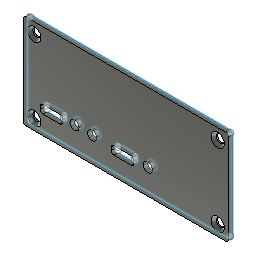
Front Plate (Autodesk Fusion 360 design; units mm, degrees)
Autodesk Fusion 360 part; units mm, degrees
sketch "sketch 658" plane through (0, 0, 0) normal (0, -1, 0) x (1, 0, 0)
  circle A0 centre (8.103, -8.2082) radius 1.7
  arc A1 (-24.375, -7.4644) -> (-23.375, -8.4644) centre (-24.375, -8.4644) cw
  line L0 (-23.375, -8.4644) -> (-23.375, -9.5644)
  arc A2 (-23.375, -9.5644) -> (-24.375, -10.5644) centre (-24.375, -9.5644) cw
  line L1 (-24.375, -10.5644) -> (-30.775, -10.5644)
  arc A3 (-30.775, -10.5644) -> (-31.775, -9.5644) centre (-30.775, -9.5644) cw
  line L2 (-31.775, -9.5644) -> (-31.775, -8.4644)
  arc A4 (-31.775, -8.4644) -> (-30.775, -7.4644) centre (-30.775, -8.4644) cw
  line L3 (-30.775, -7.4644) -> (-24.375, -7.4644)
  line L4 (-4.475, -7.5152) -> (1.925, -7.5152)
  line L5 (-4.475, -7.5152) -> (1.925, -7.5152)
  arc A5 (1.925, -7.5152) -> (2.925, -8.5152) centre (1.925, -8.5152) cw
  line L6 (2.925, -8.5152) -> (2.925, -9.6152)
  arc A6 (2.925, -9.6152) -> (1.925, -10.6152) centre (1.925, -9.6152) cw
  line L7 (1.925, -10.6152) -> (-4.475, -10.6152)
  line L8 (1.925, -10.6152) -> (-4.475, -10.6152)
  arc A7 (-4.475, -10.6152) -> (-5.475, -9.6152) centre (-4.475, -9.6152) cw
  line L9 (-5.475, -9.6152) -> (-5.475, -8.5152)
  arc A8 (-5.475, -8.5152) -> (-4.475, -7.5152) centre (-4.475, -8.5152) cw
  circle A9 centre (-19.0635, -8.2082) radius 1.7
  circle A10 centre (-12.4985, -8.2082) radius 1.7
  arc A11 (-37, 17.5) -> (-38, 16.5) centre (-37, 16.5) ccw
  line L10 (-38, 16.5) -> (-38, -16.5)
  line L11 (-38, 16.5) -> (-38, -16.5)
  arc A12 (-38, -16.5) -> (-37, -17.5) centre (-37, -16.5) ccw
  line L12 (-37, -17.5) -> (37, -17.5)
  line L13 (-37, -17.5) -> (37, -17.5)
  arc A13 (37, -17.5) -> (38, -16.5) centre (37, -16.5) ccw
  line L14 (38, -16.5) -> (38, 16.5)
  line L15 (38, -16.5) -> (38, 16.5)
  arc A14 (38, 16.5) -> (37, 17.5) centre (37, 16.5) ccw
  line L16 (37, 17.5) -> (-37, 17.5)
  line L17 (37, 17.5) -> (-37, 17.5)
extrude "Extrude1" add sketch "sketch 658" along normal blind 1.5
hole "Hole1" at (-34, -1.5, 13.5) direction (0, 1, 0) diameter 3 depth 2.75 tip angle 180 countersink diameter 5 countersink angle 90
hole "Hole2" at (-34, -1.5, -13.5) direction (0, 1, 0) diameter 3 depth 2.75 tip angle 180 countersink diameter 5 countersink angle 90
hole "Hole3" at (34, -1.5, 13.5) direction (0, 1, 0) diameter 3 depth 2.75 tip angle 180 countersink diameter 5 countersink angle 90
hole "Hole4" at (34, -1.5, -13.5) direction (0, 1, 0) diameter 3 depth 2.75 tip angle 180 countersink diameter 5 countersink angle 90
